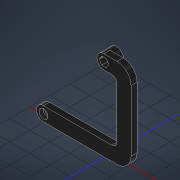
# Autodesk Inventor part: Door_Lever2
Saved by Autodesk Inventor 2022.2 (Build 262287010, 287A)
## iProperties
Created: 2022-01-24
Part Number: Door_Lever2
Material: ABS-Kunststoff
Document SubType Name: Modeling
Designer: sleib
Density: 1.06 g/cm^3
Appearance: Glatt - Schwarz
Author: sleib
Autodesk Inventor part; units mm, degrees
ref_plane "YZ Plane" through (0, 0, 0) normal (1, 0, 0) x (0, 1, 0)
ref_plane "XZ Plane" through (0, 0, 0) normal (0, 1, 0) x (-1, 0, 0)
ref_plane "XY Plane" through (0, 0, 0) normal (0, 0, 1) x (1, 0, 0)
sketch "Skizze1" plane through (0, 0, 0) normal (0, 0, 1) x (1, 0, 0)
  circle A0 centre (0, 0) radius 2.5
  line L0 (0, 7) -> (13, 7)
  arc A1 (0, 7) -> (0, -7) centre (0, 0) ccw
  circle A2 centre (-60.334, -75) radius 2.5
  line L1 (-60.334, -68) -> (8, -68)
  line L2 (13, -63) -> (13, -12)
  line L3 (27, -7) -> (27, -68)
  line L4 (13, -82) -> (-60.334, -82)
  arc A3 (-60.334, -68) -> (-60.334, -82) centre (-60.334, -75) ccw
  line L5 (20, -82) -> (20, 7) construction
  line L6 (0, 0) -> (-60.334, -75) construction
  line L7 (-60.334, -75) -> (-110.6881, -137.5941) construction
  line L8 (-60.334, -75) -> (20, -75) construction
  circle A4 centre (-60.334, -75) radius 7
  arc A5 (27, -7) -> (13, 7) centre (13, -7) ccw
  arc A6 (13, -82) -> (27, -68) centre (13, -68) ccw
  arc A7 (8, -68) -> (13, -63) centre (8, -63) ccw
  arc A8 (13, -12) -> (8, -7) centre (8, -12) ccw
  circle A9 centre (0, 0) radius 7
  line L9 (8, -7) -> (0, -7)
  line L10 (-2.3094, -4) -> (-4.6188, 0)
  line L11 (-4.6188, 0) -> (-2.3094, 4)
  line L12 (-2.3094, 4) -> (2.3094, 4)
  line L13 (2.3094, 4) -> (4.6188, 0)
  line L14 (4.6188, 0) -> (2.3094, -4)
  line L15 (2.3094, -4) -> (-2.3094, -4)
  point P0 (-60.334, -68)
  point P1 (13, 7)
  point P2 (0, -7)
  point P3 (0, -7)
  dimension "d0" = 5
  dimension "d10" = 75
  dimension "d11" = 14
  dimension "d14" = 176.5899
  dimension "d19" = 20
  dimension "d20" = 7
  dimension "d25" = 5
  dimension "d26" = 14
  dimension "d41" = 8
  constraints: 33 end point, 12 point on circle, 12 tangent, 9 centre point, 4 coincident, 4 equal radius, 4 horizontal, 4 perpendicular, 3 concentric, 3 point on line, 1 collinear, 1 equal length, 1 vertical, 18 other
  measures "d0" diameter of A0
  measures "d10" vertical distance of A2.centre point (0, 0)
  measures "d11" distance between parallel lines of L3 L2
  measures "d14" distance of L7.end point (0, 0)
  measures "d19" distance from line of L5 point (0, 0)
  measures "d20" radius of A1
  measures "d25" radius of A8
  measures "d26" radius of A6
  measures "d41" distance between parallel lines of L12 L15
extrude "Extrusion1" add sketch "Skizze1" along normal blind 6 contours A9 A1 | L0 A5 L3 A6 L4 A4 L1 A7 L2 A8 L9 A9 | A3 A4 | L10 L11 L12 L13 L14 L15
extrude "Extrusion2" add sketch "Skizze1" against normal blind 6.5 contours A9 A1 | L10 L11 L12 L13 L14 L15
sketch "Skizze2" plane through (0, 0, 6) normal (0, 0, 1) x (1, 0, 0)
  circle A0 centre (-60.334, -75) radius 2.5 projected
  circle A1 centre (0, 0) radius 2.5 projected
  constraints: 3 coincident
hole "Bohrung1" at (-60.334, -75, 6) direction (0, 0, -1) diameter 5.3 end through all counterbore diameter 9 counterbore depth 4 clearance for "Inbusschraube DIN EN ISO 4762" size "M5" standard "DIN"
sketch "Skizze3" plane through (0, 0, 6) normal (0, 0, 1) x (1, 0, 0)
  circle A0 centre (0, 0) radius 2.5 projected
  constraints: 1 coincident
hole "Bohrung2" at (0, 0, 6) direction (0, 0, -1) diameter 5.3 end through all clearance for "Inbusschraube DIN EN ISO 4762" size "M5" standard "DIN"
extrude "Extrusion3" cut sketch "Skizze1" along normal blind 6 and the other way blind 4.5 contours L10 L11 L12 L13 L14 L15
equation "\"d11\" = 2 * d20"
equation "\"d26\" = 2 * d20"
equation "\"d42\" = d6"
equation "\"d6\" = 6"
